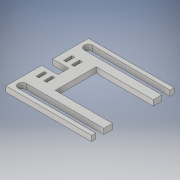
# Autodesk Inventor part: КВ33.044.204 - Держатель ремня
Saved by Autodesk Inventor 2019 (Build 230136000, 136)
## iProperties
Created: 2019-08-10
Part Number: КВ33.044.204 - Держатель ремня
Material: Типовые
Document SubType Name: Modeling
Designer: Петров Иван
Density: 1 g/cm^3
Appearance: По умолчанию
Author: Петров Иван
Autodesk Inventor part; units mm, degrees
ref_plane "YZ Plane" through (0, 0, 0) normal (1, 0, 0) x (0, 1, 0)
ref_plane "XZ Plane" through (0, 0, 0) normal (0, 1, 0) x (-1, 0, 0)
ref_plane "XY Plane" through (0, 0, 0) normal (0, 0, 1) x (1, 0, 0)
sketch "Эскиз1" plane through (0, 0, 0) normal (0, 1, 0) x (-1, 0, 0)
  line L0 (0, 0) -> (0, 24.3)
  line L1 (0, 0) -> (0, -24.3)
  line L2 (-30, 24.3) -> (30, 24.3) construction
  line L3 (-30, 21.3) -> (30, 21.3)
  line L4 (30, 27.3) -> (-30, 27.3)
  arc A0 (-30, 27.3) -> (-30, 21.3) centre (-30, 24.3) ccw
  arc A1 (30, 21.3) -> (30, 27.3) centre (30, 24.3) ccw
  line L5 (-30, -24.3) -> (30, -24.3) construction
  line L6 (-30, -27.3) -> (30, -27.3)
  line L7 (30, -21.3) -> (-30, -21.3)
  arc A2 (-30, -21.3) -> (-30, -27.3) centre (-30, -24.3) ccw
  arc A3 (30, -27.3) -> (30, -21.3) centre (30, -24.3) ccw
  line L8 (-33, 24.3) -> (-33, 30.3)
  line L9 (-33, 30.3) -> (35.9111, 30.3)
  line L10 (35.9111, 30.3) -> (35.9111, -30.3)
  line L11 (35.9111, -30.3) -> (-33, -30.3)
  line L12 (-33, -30.3) -> (-33, 30.3)
  dimension "d0" = 24.3
  dimension "d1" = 24.3
  dimension "d2" = 30
  dimension "d3" = 6
  dimension "d4" = 6
  dimension "d5" = 6
  dimension "d6" = 6
  constraints: 30 end point, 9 point on circle, 8 tangent, 4 centre point, 4 parallel, 3 vertical, 2 horizontal, 2 midpoint, 2 perpendicular
  measures "d0" distance of L0.start L0.end
  measures "d1" distance of L0.start L1.end
  measures "d2" distance of L0.end L2.end
  measures "d3" diameter of A1
  measures "d4" diameter of A3
  measures "d5" distance of L8.start L8.end
  measures "d6" distance between parallel lines of L11 L5
extrude "Выдавливание1" add sketch "Эскиз1" along normal blind 4 contours L1 L7 A2 L12 A0 L3 L0 | L0 L3 A1 L4 A0 L8 L9 L10 L11 L12 A2 L6 A3 L7 L1
sketch "Эскиз2" plane through (0, 4, 0) normal (0, 1, 0) x (1, 0, 0)
  line L0 (33, 30.3) -> (-35.9111, 30.3) projected
  line L1 (33, -30.3) -> (27, -30.3)
  line L2 (27, -30.3) -> (27, 30.3)
  line L3 (27, 30.3) -> (33, 30.3)
  line L4 (33, 30.3) -> (33, -30.3)
  point P0 (0, 0)
  dimension "d9" = 6
  constraints: 8 end point, 2 parallel, 1 horizontal, 1 perpendicular, 1 point on line
  measures "d9" distance of L2.end L3.end
extrude "Выдавливание2" cut sketch "Эскиз2" against normal through all
sketch "Эскиз3" plane through (0, 4, 0) normal (0, 1, 0) x (1, 0, 0)
  line L0 (27, 21.3) -> (27, -21.3) projected
  line L1 (27, 0) -> (27, -15)
  line L2 (27, -15) -> (27, 15)
  line L3 (27, -15) -> (-4.4812, -15)
  line L4 (-4.4812, -15) -> (-4.4812, 15)
  line L5 (-4.4812, 15) -> (27, 15)
  line L6 (27, 15) -> (27, -15)
  point P0 (0, 0)
  dimension "d12" = 15
  dimension "d13" = 30
  constraints: 12 end point, 2 parallel, 2 point on line, 1 horizontal, 1 midpoint, 1 perpendicular
  measures "d12" distance of L1.start L1.end
  measures "d13" distance of L1.end L2.end
extrude "Выдавливание3" cut sketch "Эскиз3" against normal blind 4
move faces "Перенос1" translate (-10.5, 0, 0) faces at (-4.4812, 2.6667, -5) (-21.4937, 0, 5)
sketch "Эскиз5" plane through (0, 4, 0) normal (0, 1, 0) x (1, 0, 0)
  line L0 (-35.9111, 30.3) -> (-35.9111, -30.3) projected
  line L1 (27, -15) -> (-14.9812, -15) projected
  line L2 (-35.9111, 15.0973) -> (-14.9812, 15.0973)
  line L3 (-14.9812, 15.0973) -> (-14.9812, -15)
  line L4 (-14.9812, -15) -> (-35.9111, -15)
  line L5 (-35.9111, -15) -> (-35.9111, 15.0973)
  point P0 (0, 0)
  constraints: 8 end point, 2 parallel, 1 horizontal, 1 perpendicular, 1 point on line
extrude "Выдавливание5" [suppressed]
sketch "Эскиз6" plane through (-35.9111, 0, 30.3) normal (0, -1, 0) x (1, 0, 0)
  line L0 (0, -45.3973) -> (20.9298, -45.3973) projected
  line L1 (0, -45.3973) -> (0, -42.3973)
  line L2 (0, -45.3973) -> (0, -15.3) projected
  line L3 (0, -15.3) -> (0, -18.3)
  line L4 (0, -42.3973) -> (15.1843, -42.3973)
  line L5 (15.1843, -42.3973) -> (15.1843, -18.3)
  line L6 (15.1843, -18.3) -> (0, -18.3)
  line L7 (0, -18.3) -> (0, -42.3973)
  point P0 (35.9111, -30.3)
  dimension "d26" = 3
  dimension "d27" = 3
  constraints: 12 end point, 2 parallel, 2 point on line, 1 horizontal, 1 perpendicular
  measures "d26" distance of L0.start L1.end
  measures "d27" distance of L2.end L3.end
extrude "Выдавливание6" [suppressed]
chamfer "Фаска1" [suppressed]
sketch "Эскиз7" plane through (0, 4, 0) normal (0, 1, 0) x (1, 0, 0)
  line L0 (-30.9111, -13.106) -> (-28.9111, -13.106)
  line L1 (-28.9111, -13.106) -> (-28.9111, -7.106)
  line L2 (-28.9111, -7.106) -> (-30.9111, -7.106)
  line L3 (-30.9111, -7.106) -> (-30.9111, -13.106)
  line L4 (-25.2291, -13.106) -> (-23.2291, -13.106)
  line L5 (-23.2291, -13.106) -> (-23.2291, -7.106)
  line L6 (-23.2291, -7.106) -> (-25.2291, -7.106)
  line L7 (-25.2291, -7.106) -> (-25.2291, -13.106)
  line L8 (0, 0) -> (-7.2083, 0)
  line L9 (-35.9111, 30.3) -> (-35.9111, -30.3) projected
  line L10 (-30.9111, 13.106) -> (-28.9111, 13.106)
  line L11 (-28.9111, 13.106) -> (-28.9111, 7.106)
  line L12 (-28.9111, 7.106) -> (-30.9111, 7.106)
  line L13 (-30.9111, 7.106) -> (-30.9111, 13.106)
  line L14 (-25.2291, 13.106) -> (-23.2291, 13.106)
  line L15 (-23.2291, 13.106) -> (-23.2291, 7.106)
  line L16 (-23.2291, 7.106) -> (-25.2291, 7.106)
  line L17 (-25.2291, 7.106) -> (-25.2291, 13.106)
  dimension "d33" = 2
  dimension "d34" = 6
  dimension "d35" = 2
  dimension "d36" = 5
  constraints: 34 end point, 8 symmetric about line, 4 parallel, 4 point on line, 3 horizontal, 2 perpendicular
  measures "d33" distance of L2.end L1.end
  measures "d34" distance of L1.end L0.end
  measures "d35" distance of L6.end L5.end
  measures "d36" distance between parallel lines of L9 L3
extrude "Выдавливание7" cut sketch "Эскиз7" against normal blind 10
sketch "Эскиз8" plane through (0, 4, 0) normal (0, 1, 0) x (1, 0, 0)
  line L0 (-35.9111, 30.3) -> (-35.9111, -30.3) projected
  line L1 (-35.9111, 0) -> (-35.9111, -4)
  line L2 (-35.9111, -4) -> (-25.9111, -4)
  line L3 (-35.9111, -4) -> (-23.9111, -4)
  line L4 (-23.9111, -4) -> (-23.9111, 4)
  line L5 (-23.9111, 4) -> (-35.9111, 4)
  line L6 (-35.9111, 4) -> (-35.9111, -4)
  point P0 (0, 0)
  dimension "d39" = 4
  dimension "d40" = 10
  dimension "d41" = 12
  dimension "d42" = 8
  constraints: 12 end point, 2 parallel, 2 perpendicular, 1 horizontal, 1 midpoint, 1 point on line
  measures "d39" distance of L1.start L1.end
  measures "d40" distance of L1.end L2.end
  measures "d41" distance of L5.end L4.end
  measures "d42" distance of L4.end L3.end
extrude "Выдавливание8" cut sketch "Эскиз8" against normal blind 10
